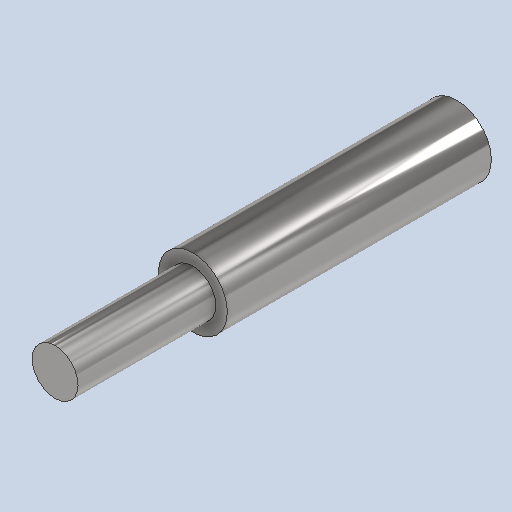
# Autodesk Inventor part: crank_shaft
Saved by Autodesk Inventor 2022.2 (Build 262287010, 287A)
## iProperties
Created: 2022-05-04
Part Number: crank_shaft
Material: Steel, Mild
Document SubType Name: Modeling
Designer: 19710060
Density: 7.85 g/cm^3
Appearance: Semi-Polished
Author: 19710060
Autodesk Inventor part; units mm, degrees
ref_plane "YZ Plane" through (0, 0, 0) normal (1, 0, 0) x (0, 1, 0)
ref_plane "XZ Plane" through (0, 0, 0) normal (0, 1, 0) x (-1, 0, 0)
ref_plane "XY Plane" through (0, 0, 0) normal (0, 0, 1) x (1, 0, 0)
sketch "Esboço1" plane through (0, 0, 0) normal (1, 0, 0) x (0, 1, 0)
  line L0 (0, 0) -> (2, 0)
  line L1 (2, 0) -> (2, -12)
  line L2 (2, -12) -> (3, -12)
  line L3 (3, -12) -> (3, -35)
  line L4 (3, -35) -> (0, -35)
  line L5 (0, -35) -> (0, 0)
  dimension "d0" = 2
  dimension "d1" = 12
  dimension "d2" = 1
  dimension "d3" = 23
  constraints: 12 end point, 5 perpendicular, 1 horizontal
  measures "d0" distance of L0.start L0.end
  measures "d1" distance of L0.end L1.end
  measures "d2" distance of L1.end L2.end
  measures "d3" distance of L2.end L3.end
revolve "Revolução1" add sketch "Esboço1" angle 360 about axis through (0, 0, -35) along (0, 0, 1)
